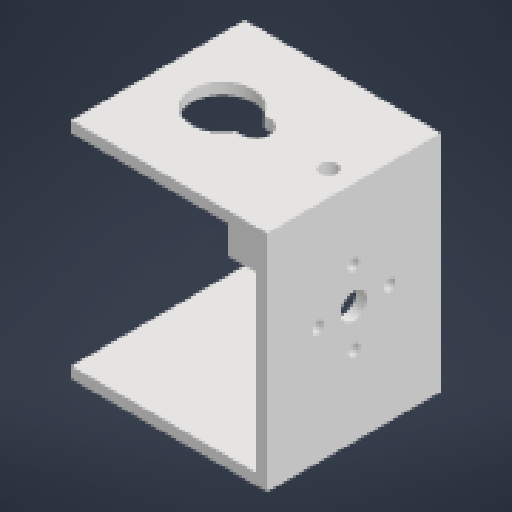
# Autodesk Inventor part: Part4
Saved by Autodesk Inventor 2024.2 (Build 282272000, 272)
## iProperties
Created: 2024-03-20
Part Number: Part4
Material: Generic
Document SubType Name: Modeling
Designer: seifs
Density: 1 g/cm^3
Appearance: Default
Author: seifs
Autodesk Inventor part; units mm, degrees
ref_plane "YZ Plane" through (0, 0, 0) normal (1, 0, 0) x (0, 1, 0)
ref_plane "XZ Plane" through (0, 0, 0) normal (0, 1, 0) x (-1, 0, 0)
ref_plane "Work Plane1" through (0, 0, 0) normal (0, 0, 1) x (1, 0, 0)
sketch "Sketch1" plane through (0, 0, 0) normal (0, 0, 1) x (1, 0, 0)
  line L0 (27, 15) -> (27, 17) projected
  line L1 (21.5, 17) -> (26.5, 17) construction
  line L2 (22, 17) -> (22, 21.5) projected
  line L3 (27, 15) -> (27, 17) projected
  line L4 (21.5, 17) -> (26.5, 17) projected
  line L5 (21.5, 22) -> (7.7913, 22) projected
  line L6 (14, 22) -> (14, 26.5) construction
  line L7 (27, 15) -> (27, 17)
  line L8 (22, 17) -> (27, 17)
  line L9 (22, 17) -> (22, 21.5)
  line L10 (21.5, 22) -> (22, 22)
  line L11 (22, 22) -> (22, 21.5)
  line L12 (21.5, 22) -> (14, 22)
  line L13 (11.5, 27) -> (13.5, 27) projected
  line L14 (7.7913, 22) -> (21.5, 22) projected
  line L15 (27, 15) -> (27, 0)
  line L16 (14, 22) -> (14, 24)
  line L17 (14, 24) -> (27, 24)
  line L18 (27, 24) -> (29, 24)
  line L19 (29, -16) -> (29, 24)
  line L20 (29, -16) -> (-6, -16)
  line L21 (-6, -16) -> (-6, -14)
  line L22 (-6, -14) -> (27, -14)
  line L23 (27, -14) -> (27, 0)
  point P0 (0, 0)
  dimension "d0" = 2
  dimension "d1" = 2
  dimension "d2" = 40
  dimension "d3" = 35
  dimension "d4" = 2
  constraints: 32 end point, 7 perpendicular, 3 point on line, 2 collinear, 2 horizontal, 2 vertical, 2 other
  measures "d0" distance of L6.start L16.end
  measures "d1" distance of L17.end L18.end
  measures "d2" distance of L19.start L18.end
  measures "d3" distance of L19.start L20.end
  measures "d4" distance of L20.end L21.end
extrude "Extrusion1" add sketch "Sketch1" along normal blind 10 and the other way blind 21
sketch "Sketch2" plane through (14, 24, 10) normal (0, 1, 0) x (1, 0, 0)
  arc A0 (-3.601, 18) -> (-3.601, 13) centre (-8.5, 15.5) ccw projected
  arc A1 (-3.601, 18) -> (-3.601, 13) centre (-8.5, 15.5) ccw
  arc A2 (-2.5, 13) -> (-2.5, 18) centre (-2.5, 15.5) ccw projected
  line L0 (-2.5, 13) -> (-3.601, 13) projected
  line L1 (-2.5, 18) -> (-3.601, 18) projected
  arc A3 (-2.5, 13) -> (-2.5, 18) centre (-2.5, 15.5) ccw
  line L2 (-3.601, 13) -> (-2.5, 13)
  line L3 (-3.601, 18) -> (-2.5, 18)
  line L4 (0.5, 15.5) -> (0.5, 0)
  line L5 (15, 0) -> (0, 0) projected
  line L6 (0.5, 15.5) -> (0.5, 31)
  line L7 (0, 31) -> (0, 0) projected
  line L8 (13, 0) -> (-20, 0) projected
  line L9 (0.5, 0) -> (-20, 0)
  line L10 (-20, 31) -> (-20, 0) projected
  line L11 (-20, 0) -> (-20, 31)
  line L12 (-20, 31) -> (0.5, 31)
  point P0 (-14, 10)
  point P1 (0, 15.5)
  constraints: 17 end point, 4 point on circle, 2 centre point, 2 coincident, 2 collinear, 2 parallel, 2 perpendicular, 1 concentric, 1 point on line, 1 vertical
extrude "Extrusion2" add sketch "Sketch2" against normal blind 2 contours L7 L8 L10 L12
sketch "Sketch3" plane through (22, 17, 10) normal (0, -1, 0) x (1, 0, 0)
  arc A0 (3.799, -14.75) -> (3.799, -16.25) centre (2.5, -15.5) ccw projected
  circle A1 centre (2.5, -15.5) radius 1.5
  point P0 (-22, -10)
  point P1 (3.799, -16.25)
  point P2 (3.799, -14.75)
  constraints: 1 centre point, 1 coincident, 1 concentric
extrude "Extrusion3" cut sketch "Sketch3" against normal blind 17
sketch "Sketch4" plane through (29, -16, 10) normal (1, 0, 0) x (0, 0, -1)
  line L0 (13, 40) -> (18, 40) projected
  line L1 (15.5, 40) -> (15.5, 21)
  circle A0 centre (15.5, 21) radius 2.3
  point P0 (10, 16)
  dimension "d15" = 19
  dimension "d16" = 4.6
  constraints: 2 end point, 1 centre point, 1 coincident, 1 midpoint, 1 vertical
  measures "d15" distance of L1.start L1.end
  measures "d16" diameter of A0
extrude "Extrusion4" cut sketch "Sketch4" against normal blind 2
sketch "Sketch5" plane through (29, -16, 10) normal (1, 0, 0) x (0, 0, -1)
  circle A0 centre (21.9497, 21.0658) radius 0.6
  circle A1 centre (9.0503, 20.9342) radius 0.6
  circle A2 centre (15.4342, 27.4497) radius 0.6
  circle A3 centre (15.5699, 14.1504) radius 0.6
  circle A4 centre (15.4342, 27.4497) radius 1
  circle A5 centre (21.9497, 21.0658) radius 1
  circle A6 centre (15.5699, 14.1504) radius 1
  circle A7 centre (9.0503, 20.9342) radius 1
  point P0 (10, 16)
  dimension "d19" = 2
  dimension "d20" = 2
  dimension "d21" = 2
  dimension "d22" = 2
  constraints: 8 centre point, 4 coincident, 8 other
  measures "d19" diameter of A4
  measures "d20" diameter of A5
  measures "d21" diameter of A6
  measures "d22" diameter of A7
extrude "Extrusion5" cut sketch "Sketch5" against normal blind 2.1 contours A0 | A1 | A3 | A5 | A6 | A7
fillet "Fillet1" radius 2 4 edges at (27, -14, -5.5) (22, 17, -5.5) (29, 24, -5.5) (29, -16, -5.5)
fillet "Fillet2" radius 2 2 edges at (-6, -16, -5.5) (-6, 24, -5.5)
sketch "Sketch6" plane through (27, -16, -21) normal (0, -1, 0) x (1, 0, 0)
  circle A0 centre (-21.5, 15.5) radius 1.5
  circle A1 centre (-21.5, 15.5) radius 1.5
  point P0 (-27, 21)
  constraints: 2 centre point, 1 coincident, 1 concentric, 2 other
extrude "Extrusion6" cut sketch "Sketch6" against normal blind 3
body "Solid1"
